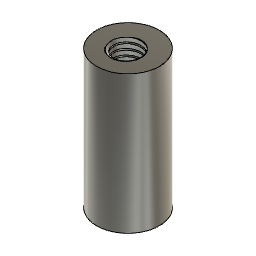
Standoff Spacer v1 v1 (Autodesk Fusion 360 design; units mm, degrees)
Autodesk Fusion 360 part; units mm, degrees
sketch "Sketch1" plane through (0, 0, 0) normal (0, 0, 1) x (1, 0, 0) in component "Standoff Spacer"
  circle A0 centre (0, 0) radius 2.5
  dimension "d3" = 5
  constraint coincident A0.centre origin
  measures "d3" diameter of A0
extrude "Extrude1" add sketch "Sketch1" along normal blind 11 in component "Standoff Spacer"
hole "Hole1" at (0, 0, 11) direction (0, 0, -1) diameter 2.175 depth 11 tip angle 180 in component "Standoff Spacer"
thread "Thread1" "ISO Metric profile 2.6 M2.6x0.45 6H" major diameter 2.675 minor diameter 2.1754 pitch 0.45 angle 60 modelled right hand crest width 0.1241 on face at (0.0542, -1.0861, 7.3333) crest through (1.0877, 0, 10.8875) in component "Standoff Spacer"
component "Standoff Spacer" placed x (1, 0, 0) y (0, 1, 0) z (0, 0, 1) at (0, 0, 0)
equation "StandoffHeight = 11 mm"
equation "StandoffWidth = 5 mm"
equation "d3 = StandoffWidth"
equation "d4 = StandoffHeight"
equation "d6 = StandoffHeight"
